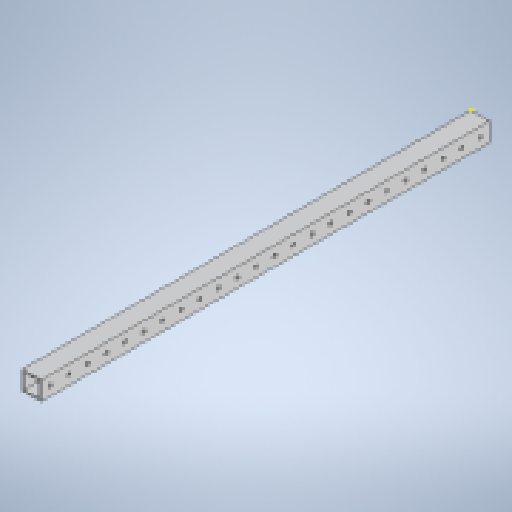
# Autodesk Inventor part: Leg_tube
Saved by Autodesk Inventor 2024 (Build 280153000, 153)
## iProperties
Created: 2023-04-20
Part Number: Leg_tube
Material: Generic
Document SubType Name: Modeling
Designer: legom
Density: 1 g/cm^3
Appearance: Default
Author: legom
Autodesk Inventor part; units mm, degrees
ref_plane "YZ Plane" through (0, 0, 0) normal (1, 0, 0) x (0, 1, 0)
ref_plane "XZ Plane" through (0, 0, 0) normal (0, 1, 0) x (-1, 0, 0)
ref_plane "XY Plane" through (0, 0, 0) normal (0, 0, 1) x (1, 0, 0)
sketch "Sketch2" plane through (0, 0, 0) normal (0, 0, 1) x (1, 0, 0)
  line L0 (0, 0) -> (25.4, 0)
  line L1 (25.4, 0) -> (25.4, 25.4)
  line L2 (25.4, 25.4) -> (0, 25.4)
  line L3 (0, 25.4) -> (0, 0)
  line L4 (23.114, 23.114) -> (23.114, 2.286)
  line L5 (23.114, 2.286) -> (2.286, 2.286)
  line L6 (2.286, 2.286) -> (2.286, 23.114)
  line L7 (2.286, 23.114) -> (23.114, 23.114)
  dimension "d0" = 25.4
  dimension "d1" = 25.4
  dimension "d2" = 2.286
  constraints: 16 end point, 4 parallel, 2 perpendicular, 1 horizontal, 3 other
  measures "d0" distance of L2.end L1.end
  measures "d1" distance of L1.end L0.end
  measures "d2" distance between parallel lines of L1 L4
extrude "Extrusion1" add sketch "Sketch2" along normal blind 635
sketch "Sketch3" plane through (25.4, 0, 0) normal (1, 0, 0) x (0, 0, -1)
  circle A0 centre (-12.7, 12.7) radius 2.5527
  line L0 (0, 0) -> (-635, 0) projected
  line L1 (0, 0) -> (0, 25.4) projected
  dimension "d5" = 5.1054
  dimension "d6" = 12.7
  dimension "d7" = 12.7
  constraints: 1 centre point
  measures "d5" diameter of A0
  measures "d6" distance from line of L0 A0.centre
  measures "d7" distance from line of L1 A0.centre
extrude "Extrusion2" cut sketch "Sketch3" against normal blind 609.6
pattern_linear "Rectangular Pattern1" count 25 spacing 25.4 along (0, 0, 1) of "Extrusion2"
sketch "Sketch4" plane through (0, 25.4, 0) normal (0, 1, 0) x (1, 0, 0)
  point P0 (0, 0)
sketch "Sketch5" plane through (0, 25.4, 0) normal (0, 1, 0) x (1, 0, 0)
  circle A0 centre (12.7, -12.7) radius 4.7625
  line L0 (25.4, 0) -> (0, 0) projected
  line L1 (0, 0) -> (0, -635) projected
  circle A1 centre (12.7, -116.078) radius 4.7625
  circle A2 centre (12.7, -622.3) radius 4.7625
  circle A3 centre (12.7, -518.922) radius 4.7625
  line L2 (25.4, -635) -> (0, -635) projected
  line L3 (25.4, 0) -> (25.4, -635) projected
  point P0 (12.7, 0)
  dimension "d13" = 12.7
  dimension "d14" = 12.7
  dimension "d15" = 9.525
  dimension "d16" = 9.525
  dimension "d17" = 103.378
  dimension "d18" = 12.7
  dimension "d19" = 9.525
  dimension "d20" = 9.525
  dimension "d21" = 103.378
  dimension "d22" = 12.7
  dimension "d23" = 12.7
  dimension "d24" = 12.7
  constraints: 4 centre point, 1 midpoint
  measures "d13" distance of point (12.7, 0) A0.centre
  measures "d14" distance from line of A0.centre L1
  measures "d15" diameter of A0
  measures "d16" diameter of A1
  measures "d17" distance of A0.centre A1.centre
  measures "d18" distance from line of L1 A1.centre
  measures "d19" diameter of A2
  measures "d20" diameter of A3
  measures "d21" distance of A3.centre A2.centre
  measures "d22" distance from line of A2.centre L2
  measures "d23" distance from line of L3 A2.centre
  measures "d24" distance from line of L3 A3.centre
extrude "Extrusion3" cut sketch "Sketch5" against normal blind 635 contours A0 | A1 | A2 | A3
body "Solid1"
